Autodesk Inventor part; units mm, degrees
(part 2 of 2)
  line L862 (-47.3488, 216.5039) -> (-50.0217, 219.1769)
  line L863 (-50.0217, 226.1442) -> (-52.7477, 228.8702)
  line L864 (-47.3488, 228.8171) -> (-50.0217, 226.1442)
  line L865 (-52.7477, 228.8702) -> (-47.3488, 228.8171) construction
  line L866 (-52.7477, 228.8702) -> (-50.0748, 231.5431)
  line L867 (-50.0217, 226.1442) -> (-50.0748, 231.5431) construction
  line L868 (-50.0748, 231.5431) -> (-47.3488, 228.8171)
  line L869 (-50.0217, 219.1769) -> (-50.0748, 213.7779) construction
  line L870 (-50.0748, 207.7431) -> (-47.3488, 205.0171)
  line L871 (-50.0217, 202.3442) -> (-50.0748, 207.7431) construction
  line L872 (-52.7477, 205.0702) -> (-50.0748, 207.7431)
  line L873 (-47.3488, 205.0171) -> (-50.0217, 202.3442)
  line L874 (-52.7477, 205.0702) -> (-47.3488, 205.0171) construction
  line L875 (-50.0217, 202.3442) -> (-52.7477, 205.0702)
  line L876 (-38.0237, 249.9442) -> (-35.2976, 252.6702)
  line L877 (-40.6966, 252.6171) -> (-38.0237, 249.9442)
  line L878 (-35.2976, 252.6702) -> (-37.9706, 255.3431)
  line L879 (-37.9706, 255.3431) -> (-40.6966, 252.6171)
  line L880 (-35.2976, 264.0508) -> (-37.9706, 261.3779)
  line L881 (-37.9706, 261.3779) -> (-40.6966, 264.1039)
  line L882 (-38.0237, 266.7769) -> (-35.2976, 264.0508)
  line L883 (-40.6966, 264.1039) -> (-38.0237, 266.7769)
  line L884 (-38.0237, 273.7442) -> (-35.2976, 276.4702)
  line L885 (-37.9706, 279.1431) -> (-40.6966, 276.4171)
  line L886 (-35.2976, 276.4702) -> (-37.9706, 279.1431)
  line L887 (-37.9706, 285.1779) -> (-40.6966, 287.9039)
  line L888 (-35.2976, 287.8508) -> (-37.9706, 285.1779)
  line L889 (-40.6966, 287.9039) -> (-38.0237, 290.5769)
  line L890 (-38.0237, 290.5769) -> (-35.2976, 287.8508)
  line L891 (-40.6966, 276.4171) -> (-38.0237, 273.7442)
  line L892 (-40.6966, 205.0171) -> (-38.0237, 202.3442)
  line L893 (-38.0237, 202.3442) -> (-35.2976, 205.0702)
  line L894 (-35.2976, 205.0702) -> (-37.9706, 207.7431)
  line L895 (-37.9706, 213.7779) -> (-40.6966, 216.5039)
  line L896 (-35.2976, 216.4508) -> (-37.9706, 213.7779)
  line L897 (-40.6966, 216.5039) -> (-38.0237, 219.1769)
  line L898 (-38.0237, 219.1769) -> (-35.2976, 216.4508)
  line L899 (-37.9706, 207.7431) -> (-40.6966, 205.0171)
  line L900 (-37.9706, 237.5779) -> (-40.6966, 240.3039)
  line L901 (-40.6966, 240.3039) -> (-38.0237, 242.9769)
  line L902 (-35.2976, 240.2508) -> (-37.9706, 237.5779)
  line L903 (-38.0237, 242.9769) -> (-35.2976, 240.2508)
  line L904 (-37.9706, 231.5431) -> (-40.6966, 228.8171)
  line L905 (-40.6966, 228.8171) -> (-38.0237, 226.1442)
  line L906 (-35.2976, 228.8702) -> (-37.9706, 231.5431)
  line L907 (-38.0237, 226.1442) -> (-35.2976, 228.8702)
  line L908 (-28.9477, 252.6702) -> (-26.2748, 255.3431)
  line L909 (-26.2217, 249.9442) -> (-28.9477, 252.6702)
  line L910 (-23.5488, 252.6171) -> (-26.2217, 249.9442)
  line L911 (-26.2748, 255.3431) -> (-23.5488, 252.6171)
  line L912 (-28.9477, 264.0508) -> (-26.2748, 261.3779)
  line L913 (-26.2217, 266.7769) -> (-28.9477, 264.0508)
  line L914 (-23.5488, 264.1039) -> (-26.2217, 266.7769)
  line L915 (-26.2748, 261.3779) -> (-23.5488, 264.1039)
  line L916 (-26.2748, 279.1431) -> (-23.5488, 276.4171)
  line L917 (-26.2217, 273.7442) -> (-28.9477, 276.4702)
  line L918 (-28.9477, 276.4702) -> (-26.2748, 279.1431)
  line L919 (-23.5488, 276.4171) -> (-26.2217, 273.7442)
  line L920 (-28.9477, 287.8508) -> (-26.2748, 285.1779)
  line L921 (-26.2217, 290.5769) -> (-28.9477, 287.8508)
  line L922 (-26.2748, 285.1779) -> (-23.5488, 287.9039)
  line L923 (-23.5488, 287.9039) -> (-26.2217, 290.5769)
  line L924 (-28.9477, 240.2508) -> (-26.2748, 237.5779)
  line L925 (-26.2748, 237.5779) -> (-23.5488, 240.3039)
  line L926 (-26.2217, 242.9769) -> (-28.9477, 240.2508)
  line L927 (-23.5488, 240.3039) -> (-26.2217, 242.9769)
  line L928 (-26.2748, 213.7779) -> (-23.5488, 216.5039)
  line L929 (-28.9477, 216.4508) -> (-26.2748, 213.7779)
  line L930 (-26.2217, 219.1769) -> (-28.9477, 216.4508)
  line L931 (-23.5488, 216.5039) -> (-26.2217, 219.1769)
  line L932 (-28.9477, 205.0702) -> (-26.2748, 207.7431)
  line L933 (-26.2748, 207.7431) -> (-23.5488, 205.0171)
  line L934 (-26.2217, 202.3442) -> (-28.9477, 205.0702)
  line L935 (-23.5488, 205.0171) -> (-26.2217, 202.3442)
  line L936 (-28.9477, 228.8702) -> (-26.2748, 231.5431)
  line L937 (-26.2748, 231.5431) -> (-23.5488, 228.8171)
  line L938 (-23.5488, 228.8171) -> (-26.2217, 226.1442)
  line L939 (-26.2217, 226.1442) -> (-28.9477, 228.8702)
  line L940 (-11.4976, 252.6702) -> (-14.1706, 255.3431)
  line L941 (-14.1706, 255.3431) -> (-16.8966, 252.6171)
  line L942 (-14.2237, 249.9442) -> (-11.4976, 252.6702)
  line L943 (-16.8966, 252.6171) -> (-14.2237, 249.9442)
  line L944 (-14.1706, 261.3779) -> (-16.8966, 264.1039)
  line L945 (-16.8966, 264.1039) -> (-14.2237, 266.7769)
  line L946 (-14.2237, 266.7769) -> (-11.4976, 264.0508)
  line L947 (-11.4976, 264.0508) -> (-14.1706, 261.3779)
  line L948 (-16.8966, 276.4171) -> (-14.2237, 273.7442)
  line L949 (-14.1706, 279.1431) -> (-16.8966, 276.4171)
  line L950 (-11.4976, 276.4702) -> (-14.1706, 279.1431)
  line L951 (-14.2237, 273.7442) -> (-11.4976, 276.4702)
  line L952 (-16.8966, 287.9039) -> (-14.2237, 290.5769)
  line L953 (-14.1706, 285.1779) -> (-16.8966, 287.9039)
  line L954 (-14.2237, 290.5769) -> (-11.4976, 287.8508)
  line L955 (-11.4976, 287.8508) -> (-14.1706, 285.1779)
  line L956 (-11.4976, 240.2508) -> (-14.1706, 237.5779)
  line L957 (-14.2237, 242.9769) -> (-11.4976, 240.2508)
  line L958 (-16.8966, 240.3039) -> (-14.2237, 242.9769)
  line L959 (-14.1706, 237.5779) -> (-16.8966, 240.3039)
  line L960 (-11.4976, 228.8702) -> (-14.1706, 231.5431)
  line L961 (-14.1706, 231.5431) -> (-16.8966, 228.8171)
  line L962 (-14.2237, 226.1442) -> (-11.4976, 228.8702)
  line L963 (-16.8966, 228.8171) -> (-14.2237, 226.1442)
  line L964 (-11.4976, 216.4508) -> (-14.1706, 213.7779)
  line L965 (-14.1706, 213.7779) -> (-16.8966, 216.5039)
  line L966 (-14.2237, 219.1769) -> (-11.4976, 216.4508)
  line L967 (-16.8966, 216.5039) -> (-14.2237, 219.1769)
  line L968 (-11.4976, 205.0702) -> (-14.1706, 207.7431)
  line L969 (-14.1706, 207.7431) -> (-16.8966, 205.0171)
  line L970 (-16.8966, 205.0171) -> (-14.2237, 202.3442)
  line L971 (-14.2237, 202.3442) -> (-11.4976, 205.0702)
  point P0 (0, 0)
  point P1 (-50.0482, 14.6436)
  point P2 (-50.0482, 26.0774)
  point P3 (-50.0482, 49.8774)
  point P4 (-50.0482, 38.4436)
  point P5 (-50.0482, 97.4774)
  point P6 (-50.0482, 86.0436)
  point P7 (-50.0482, 73.6774)
  point P8 (-50.0482, 62.2436)
  point P9 (-50.0482, 192.6774)
  point P10 (-50.0482, 181.2436)
  point P11 (-50.0482, 168.8774)
  point P12 (-50.0482, 157.4436)
  point P13 (-50.0482, 109.8436)
  point P14 (-50.0482, 145.0774)
  point P15 (-50.0482, 133.6436)
  point P16 (-50.0482, 121.2774)
  point P17 (-50.0482, 300.2436)
  point P18 (-50.0482, 264.0774)
  point P19 (-50.0482, 276.4436)
  point P20 (-50.0482, 287.8774)
  point P21 (-50.0482, 252.6436)
  point P22 (-50.0482, 240.2774)
  point P23 (-50.0482, 216.4774)
  point P24 (-50.0482, 228.8436)
  point P25 (-50.0482, 205.0436)
  dimension "d4" = 4.572
  dimension "d5" = 4.572
  dimension "d8" = 11.9
  dimension "d11" = 11.9
  constraints: 1944 end point, 153 symmetric about line, 52 midpoint, 4 parallel, 2 collinear, 2 horizontal, 2 perpendicular, 1 vertical, 1030 other
  measures "d4" distance of L2.end L1.end
  measures "d5" distance of L1.end L0.end
  measures "d8" distance of L2.end L4.start
  measures "d11" distance of L2.end L104.start
extrude "Extrusion2" cut sketch "Sketch2" against normal through all
body "Solid1"
